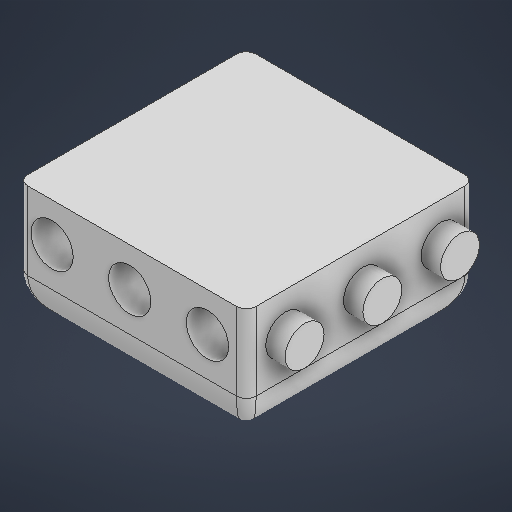
# Autodesk Inventor part: base_support
Saved by Autodesk Inventor 2026.1 (Build 301233020, 233B)
## iProperties
Created: 2025-10-30
Part Number: base_support
Material: Generic
Document SubType Name: Modeling
Designer: Asus
Density: 1 g/cm^3
Appearance: Default
Author: Asus
Autodesk Inventor part; units mm, degrees
ref_plane "YZ Plane" through (0, 0, 0) normal (1, 0, 0) x (0, 1, 0)
ref_plane "XZ Plane" through (0, 0, 0) normal (0, 1, 0) x (-1, 0, 0)
ref_plane "XY Plane" through (0, 0, 0) normal (0, 0, 1) x (1, 0, 0)
sketch "Sketch1" plane through (0, 0, 0) normal (0, 1, 0) x (-1, 0, 0)
  line L0 (0, 0) -> (23.5, 0)
  line L1 (23.5, 0) -> (23.5, -23.5)
  line L2 (23.5, -23.5) -> (0, -23.5)
  line L3 (0, -23.5) -> (0, 0)
  dimension "d0" = 23.5
  dimension "d1" = 23.5
  constraints: 8 end point, 2 parallel, 1 horizontal, 1 perpendicular
  measures "d0" distance of L1.end L2.end
  measures "d1" distance of L0.end L1.end
extrude "Extrusion1" add sketch "Sketch1" along normal blind 8
sketch "Sketch2" plane through (0, 0, 0) normal (1, 0, 0) x (0, 0, -1)
  circle A0 centre (4, 4) radius 2
  circle A1 centre (12, 4) radius 2
  circle A2 centre (20, 4) radius 2
  line L0 (0, 0) -> (0, 8) projected
  point P0 (0, 4)
  dimension "d4" = 4
  dimension "d5" = 4
  dimension "d6" = 4
  dimension "d7" = 4
  dimension "d8" = 8
  dimension "d9" = 8
  constraints: 3 centre point, 1 midpoint
  measures "d4" diameter of A0
  measures "d5" diameter of A1
  measures "d6" diameter of A2
  measures "d7" distance of point (0, 4) A0.centre
  measures "d8" distance of A1.centre A0.centre
  measures "d9" distance of A2.centre A1.centre
extrude "Extrusion2" add sketch "Sketch2" along normal blind 2
sketch "Sketch3" plane through (-23.5, 0, 0) normal (0, 0, 1) x (1, 0, 0)
  circle A0 centre (19.5, 4) radius 2.175
  circle A1 centre (11.5, 4) radius 2.175
  circle A2 centre (3.5, 4) radius 2.175
  line L0 (23.5, 0) -> (23.5, 8) projected
  dimension "d12" = 4.35
  dimension "d13" = 4.35
  dimension "d14" = 4.35
  dimension "d15" = 4
  dimension "d16" = 8
  dimension "d17" = 8
  constraints: 3 centre point
  measures "d12" diameter of A0
  measures "d13" diameter of A1
  measures "d14" diameter of A2
  measures "d15" distance from line of L0 A0.centre
  measures "d16" distance of A0.centre A1.centre
  measures "d17" distance of A1.centre A2.centre
extrude "Extrusion3" cut sketch "Sketch3" against normal blind 27
sketch "Sketch6" plane through (0, 0, 0) normal (0, -1, 0) x (1, 0, 0)
  line L0 (-23.5, 0) -> (0, 0) projected
  line L1 (0, -23.5) -> (-23.5, -23.5) projected
  line L2 (-23.5, 0) -> (0, 0)
  line L3 (0, 0) -> (0, -23.5)
  line L4 (0, -23.5) -> (-23.5, -23.5)
  line L5 (-23.5, -23.5) -> (-23.5, 0)
  constraints: 8 end point, 2 parallel, 1 horizontal, 1 perpendicular
extrude "Extrusion5" add sketch "Sketch6" along normal blind 4.5
fillet "Fillet1" radius 4.5 4 edges at (-11.75, -4.5, 0) (0, -4.5, -11.75) (-11.75, -4.5, -23.5) (-23.5, -4.5, -11.75)
fillet "Fillet2" radius 1 8 edges at (-1.318, -3.182, -1.318) (0, 4, 0) (-1.318, -3.182, -22.182) (0, 4, -23.5) (-23.5, 4, -23.5) (-22.182, -3.182, -22.182) (-23.5, 4, 0) (-22.182, -3.182, -1.318)
body "Solid1"
